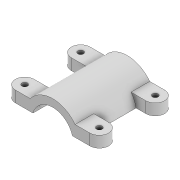
# Autodesk Inventor part: Shaft_conn_Tensioner
Saved by Autodesk Inventor 2022 (Build 260153000, 153)
## iProperties
Created: 2022-11-20
Part Number: Shaft_conn_Tensioner
Material: Generic
Document SubType Name: Modeling
Designer: MVeszpremi
Density: 1 g/cm^3
Appearance: Default
Author: MVeszpremi
Autodesk Inventor part; units mm, degrees
ref_plane "YZ Plane" through (0, 0, 0) normal (1, 0, 0) x (0, 1, 0)
ref_plane "XZ Plane" through (0, 0, 0) normal (0, 1, 0) x (-1, 0, 0)
ref_plane "XY Plane" through (0, 0, 0) normal (0, 0, 1) x (1, 0, 0)
sketch "Sketch1" plane through (0, 0, 0) normal (0, 0, 1) x (1, 0, 0)
  circle A0 centre (0, 0) radius 11
  line L0 (-10.583, 3) -> (10.583, 3)
  circle A1 centre (0, 0) radius 15
  line L1 (-14.6969, 3) -> (14.6969, 3)
  dimension "d0" = 22
  dimension "d1" = 3
  dimension "d2" = 4
  constraints: 4 end point, 4 point on circle, 2 centre point, 2 coincident, 2 point on line, 1 horizontal
  measures "d0" diameter of A0
  measures "d1" distance from line of point (0, 0) L0
  measures "d2" radial gap between concentric circles of A0 A1
extrude "Extrusion1" add sketch "Sketch1" along normal blind 40 contours A0 L1 A1 picked at (-0.4305, 13.5639)
sketch "Sketch2" plane through (10.583, 3, 0) normal (0, -1, 0) x (1, 0, 0)
  line L0 (-10.583, 0) -> (9.417, 0)
  line L1 (-10.583, 0) -> (-10.583, 40)
  line L2 (-21.166, 40) -> (0, 40) projected
  line L3 (-10.583, 20) -> (9.417, 20)
  line L4 (9.417, 20) -> (9.417, 5)
  circle A0 centre (9.417, 5) radius 1.5
  circle A1 centre (9.417, 5) radius 5
  line L5 (0, 0) -> (4.1139, 0) projected
  line L6 (9.417, 10) -> (4.1139, 10)
  line L7 (4.1139, 10) -> (4.1139, 0)
  line L8 (4.1139, 0) -> (9.417, 0)
  line L9 (9.417, 0) -> (9.417, 10)
  line L10 (-10.583, 40) -> (9.417, 40)
  circle A2 centre (9.417, 35) radius 1.5
  circle A3 centre (9.417, 35) radius 5
  line L11 (9.417, 30) -> (4.1139, 30)
  line L12 (9.417, 40) -> (9.417, 30)
  line L13 (0, 0) -> (4.1139, 0) projected
  line L14 (4.1139, 0) -> (4.1139, 40) projected
  line L15 (0, 40) -> (4.1139, 40) projected
  line L16 (0, 0) -> (0, 40) projected
  line L17 (4.1139, 30) -> (0, 30)
  line L18 (4.1139, 10) -> (0, 10)
  line L19 (0, 0) -> (0, 40) projected
  point P0 (0, 20)
  point P1 (4.1139, 20)
  dimension "d8" = 10
  dimension "d5" = 20
  dimension "d6" = 15
  dimension "d7" = 3
  constraints: 26 end point, 6 symmetric about line, 4 horizontal, 3 coincident, 3 parallel, 3 perpendicular, 3 point on line, 2 centre point, 2 midpoint, 7 other
  measures "d5" distance of L0.start L0.end
  measures "d6" distance of L3.end L4.end
  measures "d7" diameter of A0
extrude "Extrusion2" add sketch "Sketch2" against normal blind 6 contours L16 L18 L7 L0 | L7 L6 A1 L0 | L9 A0 L4 A1 | A1 L4 A0 L9 | L10 L14 L17 L16 | L10 A3 L11 L14 | L12 A2 A3 | A3 L12 A2
mirror "Mirror1" about plane through (0, 0, 0) normal (1, 0, 0) of "Extrusion2"
body "Solid1"
